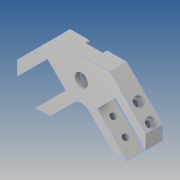
# Autodesk Inventor part: 200-20-ROCKER-CONNECTOR-03
Saved by Autodesk Inventor 2018.2 (Build 222227000, 227)
## iProperties
Manager: feesmrt
Company: FRANCOR
Part Number: 200-20-ROCKER-CONNECTOR-03
Material: Aluminium 6061
Document SubType Name: Modeling
Designer: feesmrt
Density: 2.7 g/cm^3
Appearance: Aluminium - flach
Project: Rescue Robot
Cost Center: -
Engineer: feesmrt
Authority: feesmrt
Created: 2017-12-28
Description: Rocker Profile Connector 90°
Stock Number: 200-20-ROCKER-CONNECTOR-03
Author: feesmrt
Subject: Rescue Robot
Revision Number: 1
Title: Rocker Profile Connector 90°
Autodesk Inventor part; units mm, degrees
note: some values were not read from the file. Chosen so that the rebuilt part matches the saved one: direction of "DIN7984_M6_Bohrung".
ref_plane "YZ Plane" through (0, 0, 0) normal (1, 0, 0) x (0, 1, 0)
ref_plane "XZ Plane" through (0, 0, 0) normal (0, 1, 0) x (-1, 0, 0)
sketch "Skizze1" plane through (0, 0, 0) normal (0, 1, 0) x (-1, 0, 0)
  line L0 (75, 0) -> (-5, 80) construction
  line L1 (5, 80) -> (-75, 0) construction
  line L2 (75, 21.2132) -> (39.6447, 56.5685)
  line L3 (39.6447, 56.5685) -> (18.4315, 35.3553)
  line L4 (18.4315, 35.3553) -> (53.7868, 0)
  line L5 (-18.4315, 35.3553) -> (-39.6447, 56.5685)
  line L6 (-39.6447, 56.5685) -> (-75, 21.2132)
  line L7 (-18.4315, 35.3553) -> (-53.7868, 0)
  line L8 (75, 38.1838) -> (33.1838, 80)
  line L9 (-75, 38.1838) -> (-33.1838, 80)
  line L10 (8.8388, 27.9774) -> (36.8162, 0)
  line L11 (-8.8388, 27.9774) -> (-36.8162, 0)
  arc A0 (8.8388, 27.9774) -> (-8.8388, 27.9774) centre (0, 19.1386) ccw
  line L12 (-33.1838, 80) -> (33.1838, 80)
  line L13 (53.7868, 0) -> (36.8162, 0)
  line L14 (-36.8162, 0) -> (-53.7868, 0)
  line L15 (-75, 21.2132) -> (-75, 38.1838)
  line L16 (75, 21.2132) -> (75, 38.1838)
  line L17 (0, -16) -> (0, 96) construction
  line L18 (-105, 0) -> (105, 0) construction
  line L19 (39.6447, 56.5685) -> (48.1299, 65.0538)
  point P0 (0, 36.8162)
  point P1 (0, 0)
  dimension "d11" = 30
  dimension "d12" = 50
  dimension "d16" = 12
  dimension "d17" = 12
  dimension "d18" = 12.5
  dimension "d19" = 80
  dimension "d20" = 150
  dimension "d21" = 45
  constraints: 38 end point, 12 perpendicular, 7 parallel, 6 point on line, 2 horizontal, 2 horizontal alignment, 2 point on circle, 2 tangent, 1 centre point, 1 vertical, 5 other
  measures "d11" distance of L2.end L3.end
  measures "d12" distance of L2.start L2.end
  measures "d16" distance between parallel lines of L8 L2
  measures "d17" distance between parallel lines of L4 L10
  measures "d18" radius of A0
  measures "d19" distance between parallel lines of L14 L12
  measures "d20" distance of L9.start L8.start
  measures "d21" angle to the sketch x axis of L0
extrude "Grundkörper" add sketch "Skizze1" along normal mid plane 20
sketch "Skizze2" plane through (0, 10, 0) normal (0, 1, 0) x (1, 0, 0)
  line L0 (0, 16) -> (0, -96) construction
  line L1 (-33.1838, -80) -> (33.1838, -80) construction
  line L2 (105, 0) -> (-105, 0) construction
  line L3 (10, -80) -> (-10, -80)
  line L4 (-10, -80) -> (-10, 0)
  line L5 (-10, 0) -> (10, 0)
  line L6 (10, 0) -> (10, -80)
  point P0 (0, 0)
  dimension "d25" = 20
  constraints: 8 end point, 2 parallel, 2 point on line, 1 horizontal, 1 perpendicular, 1 other
  measures "d25" distance between parallel lines of L4 L6
extrude "NUT" cut sketch "Skizze2" against normal blind 5
sketch "Skizze4" plane through (0, -10, 0) normal (0, -1, 0) x (1, 0, 0)
  line L0 (0, 96) -> (0, -16) construction
  line L1 (33.1838, 80) -> (-33.1838, 80) construction
  point P0 (0, 0)
  point P1 (0, 55)
  dimension "d29" = 25
  constraints: 1 point on line
  measures "d29" distance from line of L1 point (0, 55)
hole "DIN7984_M8_Bohrung" at (0, -10, 55) direction (0, 1, 0) diameter 9 end through all counterbore diameter 15 counterbore depth 5.4
ref_plane "Arbeitsebene_Bohrung" through (-29.0381, -10, 45.9619) normal (-0.7071068, 0, 0.7071068) x (0.7071068, 0, 0.7071068)
sketch "Skizze5" plane through (-33.1838, -10, 80) normal (-0.7071068, 0, 0.7071068) x (0.7071068, 0, 0.7071068)
  line L0 (-21.1371, 20) -> (-21.1371, 0) construction
  line L1 (-59.1371, 20) -> (-59.1371, 0) construction
  line L2 (-125.864, 10) -> (110.2244, 10) construction
  line L3 (-71.1371, 0) -> (-71.1371, 20) projected
  point P0 (-33.1041, 10)
  point P1 (-33.1371, 10)
  point P2 (-53.1371, 10)
  dimension "d37" = 20
  dimension "d39" = 18
  constraints: 2 point on line
  measures "d37" distance of point (-53.137, 10) point (-33.137, 10)
  measures "d39" distance from line of point (-53.137, 10) L3
hole "DIN7984_M6_Bohrung" at (-56.6152, 0, 56.5685) at (-70.7574, 0, 42.4264) direction (0.7071068, 0, -0.7071068) diameter 6.6 end up to surface counterbore diameter 11 counterbore depth 4.4
mirror "DIN7984_M6_Bohrung_Spiegelung:1" about plane through (-29.0381, -10, 45.9619) normal (-0.7071068, 0, 0.7071068) of "DIN7984_M6_Bohrung"
mirror "DIN7984_M6_Bohrung_Spiegelung:2" about plane through (0, 0, 0) normal (1, 0, 0) of "DIN7984_M6_Bohrung", "DIN7984_M6_Bohrung_Spiegelung:1"
equation "\"d17\" = d16"
